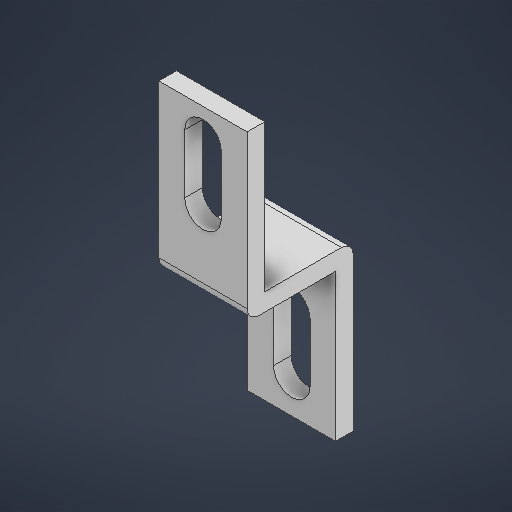
# Autodesk Inventor part: Side holding bracket
Saved by Autodesk Inventor 2027 (Build 310192000, 192)
## iProperties
Created: 2026-07-15
Part Number: Side holding bracket
Material: Generic
Document SubType Name: Modeling
Designer: ratik
Density: 1 g/cm^3
Appearance: Default
Author: ratik
Autodesk Inventor part; units mm, degrees
ref_plane "YZ Plane" through (0, 0, 0) normal (1, 0, 0) x (0, 1, 0)
ref_plane "XZ Plane" through (0, 0, 0) normal (0, 1, 0) x (-1, 0, 0)
ref_plane "XY Plane" through (0, 0, 0) normal (0, 0, 1) x (1, 0, 0)
sketch "Sketch1" plane through (0, 0, 0) normal (1, 0, 0) x (0, 1, 0)
  line L0 (47.7895, 7.9342) -> (22.7895, 7.9342)
  line L1 (22.7895, 7.9342) -> (22.7895, -7.0658)
  line L2 (22.7895, -7.0658) -> (-5.2105, -7.0658)
  line L3 (-5.2105, -7.0658) -> (-5.2105, -4.0658)
  line L4 (-5.2105, -4.0658) -> (19.7895, -4.0658)
  line L5 (19.7895, -4.0658) -> (19.7895, 10.9342)
  line L6 (19.7895, 10.9342) -> (47.7895, 10.9342)
  line L7 (47.7895, 10.9342) -> (47.7895, 7.9342)
  point P0 (0, 0)
  dimension "d0" = 3
  dimension "d1" = 3
  dimension "d2" = 3
  dimension "d3" = 15
  dimension "d4" = 25
  dimension "d5" = 25
  constraints: 16 end point, 7 perpendicular, 1 horizontal
  measures "d0" distance of L6.end L0.start
  measures "d1" distance of L2.end L3.end
  measures "d2" distance between parallel lines of L1 L5
  measures "d3" distance between parallel lines of L2 L0
  measures "d4" distance of L0.start L0.end
  measures "d5" distance of L3.end L4.end
extrude "Extrusion1" add sketch "Sketch1" along normal blind 15
fillet "Fillet1" radius 2 2 edges at (7.5, 22.7895, -7.0658) (7.5, 19.7895, 10.9342)
sketch "Sketch2" plane through (0, 47.7895, 10.9342) normal (0, 0, 1) x (1, 0, 0)
  arc A0 (10.6, -5) -> (4.4, -5) centre (7.5, -5) ccw
  line L0 (0, 0) -> (15, 0) projected
  arc A1 (4.4, -15) -> (10.6, -15) centre (7.5, -15) ccw
  line L1 (4.4, -15) -> (4.4, -5)
  line L2 (10.6, -5) -> (10.6, -15)
  line L3 (15, 0) -> (15, -26) projected
  arc A2 (10.6737, -37.1406) -> (4.4737, -37.1406) centre (7.5737, -37.1406) ccw
  line L4 (16.7377, 8.0467) -> (15.0737, 2.8292)
  arc A3 (4.4737, -47.1406) -> (10.6737, -47.1406) centre (7.5737, -47.1406) ccw
  line L5 (4.4737, -47.1406) -> (4.4737, -37.1406)
  line L6 (10.6737, -37.1406) -> (10.6737, -47.1406)
  line L7 (15.0737, 2.8292) -> (15.0737, -23.1708)
  point P0 (0, -47.7895)
  dimension "d9" = 6.2
  dimension "d10" = 5
  dimension "d11" = 6.2
  dimension "d12" = 10
  dimension "d13" = 7.5
  dimension "d15" = 7.5
  dimension "d16" = 6.2
  dimension "d17" = 5
  dimension "d18" = 6.2
  dimension "d19" = 10
  dimension "d20" = 7.5
  dimension "d21" = 7.5
  constraints: 12 end point, 8 point on circle, 6 tangent, 4 centre point
  measures "d9" diameter of A0
  measures "d10" distance from line of L0 A0.centre
  measures "d11" diameter of A1
  measures "d12" distance of L2.start L2.end
  measures "d13" distance from line of L3 A0.centre
  measures "d15" distance from line of L3 A1.centre
  measures "d16" diameter of A2
  measures "d17" distance from line of L4 A2.centre
  measures "d18" diameter of A3
  measures "d19" distance of L6.start L6.end
  measures "d20" distance from line of L7 A2.centre
  measures "d21" distance from line of L7 A3.centre
extrude "Extrusion2" cut sketch "Sketch2" against normal blind 20
body "Solid1"
